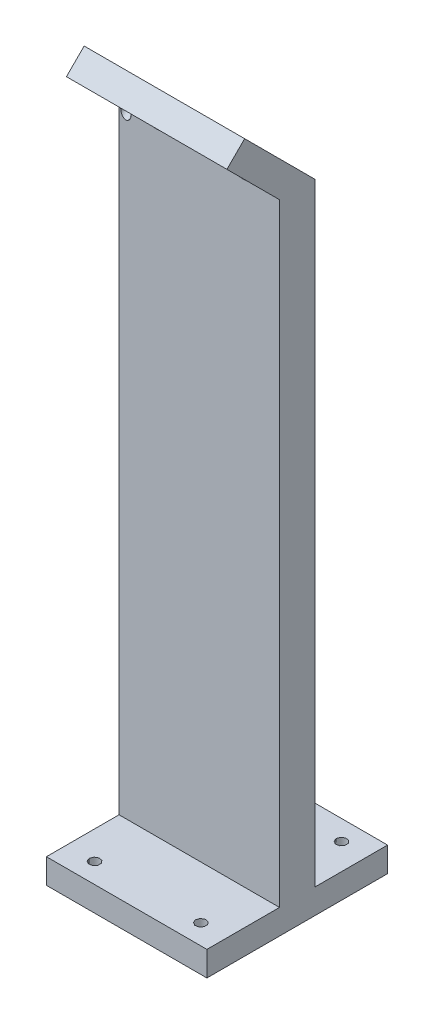
# Autodesk Inventor part: Soporte_Ultrasonido
Saved by Autodesk Inventor 2026 (Build 300175000, 175)
## iProperties
Created: 2025-06-27
Part Number: Soporte_Ultrasonido
Material: Genérico
Document SubType Name: Modeling
Designer: oscar
Density: 1 g/cm^3
Appearance: Valor por defecto
Author: oscar
Autodesk Inventor part; units mm, degrees
ref_plane "YZ Plane" through (0, 0, 0) normal (1, 0, 0) x (0, 1, 0)
ref_plane "XZ Plane" through (0, 0, 0) normal (0, 1, 0) x (-1, 0, 0)
ref_plane "XY Plane" through (0, 0, 0) normal (0, 0, 1) x (1, 0, 0)
sketch "Boceto6" plane through (0, 0, 0) normal (1, 0, 0) x (0, 1, 0)
  line L0 (0, 0) -> (180, 0)
  line L1 (180, 0) -> (180, -10)
  line L2 (180, -10) -> (0, -10)
  line L3 (0, -10) -> (0, 0)
  dimension "d12" = 180
  dimension "d13" = 10
  constraints: 8 end point, 2 parallel, 1 horizontal, 1 perpendicular
  measures "d12" distance of L1.end L2.end
  measures "d13" distance of L0.end L1.end
extrude "Extrusión3" add sketch "Boceto6" along normal mid plane 45.3
sketch "Boceto7" plane through (22.65, 0, 0) normal (1, 0, 0) x (0, 0, -1)
  line L0 (10, 0) -> (10, 180) projected
  line L1 (10, 180) -> (0, 180) projected
  line L2 (10, 180) -> (0, 180)
  line L3 (0, 180) -> (-14.8492, 194.8492)
  line L4 (10, 180) -> (-9.8492, 199.8492)
  line L5 (10, 180) -> (38.0711, 180) construction
  line L6 (-9.8492, 199.8492) -> (-14.8492, 194.8492)
  point P0 (0, 0)
  dimension "d16" = 21
  dimension "d17" = 135
  dimension "d18" = 135
  constraints: 10 end point, 2 horizontal, 1 equal length, 1 perpendicular
  measures "d16" distance of L1.end L3.end
  measures "d17" angle of L2 L3
  measures "d18" angle of L5 L4
extrude "Extrusión4" add sketch "Boceto7" against normal blind 45.3
sketch "Boceto8" plane through (22.65, 180, -10) normal (0, 0.7071, -0.7071) x (-1, 0, 0)
  circle A0 centre (10.275, 15) radius 8
  circle A1 centre (34.725, 15) radius 8
  line L0 (0, 0) -> (0, 28.0711) projected
  line L1 (45.3, 0) -> (0, 0) projected
  point P0 (22.65, -120.2082)
  dimension "d21" = 16
  dimension "d22" = 16
  dimension "d23" = 24.45
  dimension "d24" = 10.275
  dimension "d25" = 15
  dimension "d26" = 15
  constraints: 2 centre point
  measures "d21" diameter of A0
  measures "d22" diameter of A1
  measures "d23" distance of A0.centre A1.centre
  measures "d24" distance from line of L0 A0.centre
  measures "d25" distance from line of L1 A1.centre
  measures "d26" distance from line of L1 A0.centre
extrude "Extrusión5" cut sketch "Boceto8" against normal blind 8.25
sketch "Boceto11" plane through (22.65, 180, -10) normal (0, 0.7071, -0.7071) x (-1, 0, 0)
  circle A0 centre (1.95, 23.0711) radius 1.5
  line L0 (0, 0) -> (0, 28.0711) projected
  line L1 (0, 28.0711) -> (45.3, 28.0711) projected
  circle A1 centre (43.35, 7) radius 1.5
  line L2 (45.3, 28.0711) -> (45.3, 0) projected
  line L3 (45.3, 0) -> (0, 0) projected
  point P0 (22.65, -120.2082)
  point P1 (45.5, 0)
  dimension "d29" = 3
  dimension "d30" = 1.95
  dimension "d31" = 5
  dimension "d32" = 3
  dimension "d33" = 1.95
  dimension "d34" = 7
  constraints: 2 centre point, 1 other
  measures "d29" diameter of A0
  measures "d30" distance from line of L0 A0.centre
  measures "d31" distance from line of L1 A0.centre
  measures "d32" diameter of A1
  measures "d34" distance from line of L3 A1.centre
extrude "Extrusión6" cut sketch "Boceto11" against normal blind 12.5 contours A0 | A1
sketch "Boceto12" plane through (22.65, 0, -10) normal (0, 0, -1) x (-1, 0, 0)
  line L0 (0, 0) -> (0, 180) projected
  line L1 (0, 7) -> (45.3, 7)
  line L2 (45.3, 7) -> (45.3, 0)
  line L3 (45.3, 0) -> (0, 0)
  line L4 (0, 0) -> (0, 7)
  line L5 (0, 0) -> (45.3, 0) projected
  point P0 (22.65, 0)
  point P1 (22.65, 0)
  dimension "d37" = 7
  dimension "d38" = 0
  constraints: 8 end point, 2 parallel, 1 horizontal, 1 midpoint, 1 perpendicular, 1 point on line
  measures "d37" distance of L1.end L2.end
  measures "d38" distance from line of point (22.65, 0) L3
extrude "Extrusión7" add sketch "Boceto12" along normal blind 20.5
sketch "Boceto13" plane through (-22.65, 0, 0) normal (0, 0, 1) x (1, 0, 0)
  line L0 (0, 0) -> (0, 180) projected
  line L1 (0, 7) -> (45.3, 7)
  line L2 (45.3, 7) -> (45.3, 0)
  line L3 (45.3, 0) -> (0, 0)
  line L4 (0, 0) -> (0, 7)
  line L5 (0, 0) -> (45.3, 0) projected
  point P0 (22.65, 0)
  dimension "d41" = 7
  dimension "d42" = 0
  constraints: 8 end point, 2 parallel, 1 horizontal, 1 perpendicular, 1 point on line
  measures "d41" distance of L1.end L2.end
  measures "d42" distance between parallel lines of L5 L3
extrude "Extrusión8" add sketch "Boceto13" along normal blind 20.5
sketch "Boceto15" plane through (-22.65, 0, -30.5) normal (0, -1, 0) x (1, 0, 0)
  circle A0 centre (7.95, 45.3492) radius 1.5
  line L0 (45.3, 45.3492) -> (0, 45.3492) projected
  circle A1 centre (37.95, 45.3492) radius 1.5
  line L1 (0, 51) -> (45.3, 51) projected
  circle A2 centre (7.95, 5.6508) radius 1.5
  circle A3 centre (37.95, 5.6508) radius 1.5
  line L2 (45.3, 0) -> (0, 0) projected
  line L3 (45.3, 0) -> (45.3, 51) projected
  point P0 (22.65, 30.5)
  dimension "d45" = 3
  dimension "d46" = 3
  dimension "d47" = 5.6508
  dimension "d48" = 3
  dimension "d49" = 3
  dimension "d50" = 5.6508
  dimension "d51" = 5.6508
  dimension "d52" = 30
  dimension "d53" = 30
  dimension "d54" = -7.35
  dimension "d55" = -7.35
  constraints: 4 centre point, 2 point on line
  measures "d45" diameter of A0
  measures "d46" diameter of A1
  measures "d47" distance between parallel lines of L1 L0
  measures "d48" diameter of A2
  measures "d49" diameter of A3
  measures "d50" distance from line of L2 A3.centre
  measures "d51" distance from line of L2 A2.centre
  measures "d52" distance of A1.centre A0.centre
  measures "d53" distance of A3.centre A2.centre
  measures "d54" distance from line of L3 A1.centre
  measures "d55" distance from line of L3 A3.centre
extrude "Extrusión9" cut sketch "Boceto15" against normal blind 20.5
equation "\"d50\" = d47"
equation "\"d51\" = d47"
equation "\"d55\" = d54"
